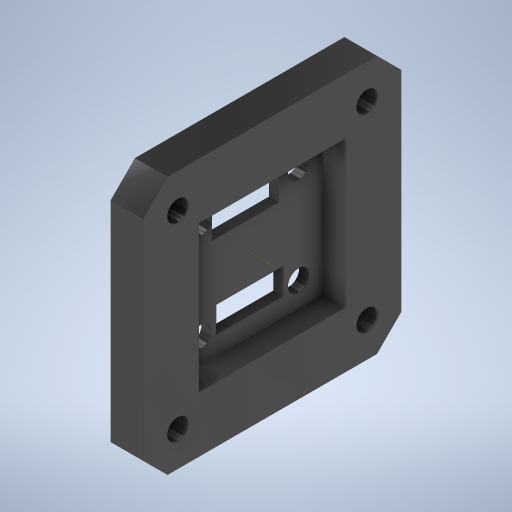
# Autodesk Inventor part: EncoderHalter
Saved by Autodesk Inventor 2023 (Build 270158000, 158)
## iProperties
Created: 2024-01-25
Part Number: EncoderHalter
Material: Generisch
Document SubType Name: Modeling
Designer: phili
Density: 1 g/cm^3
Appearance: Vorgabe
Author: phili
Autodesk Inventor part; units mm, degrees
ref_plane "YZ Plane" through (0, 0, 0) normal (1, 0, 0) x (0, 1, 0)
ref_plane "XZ Plane" through (0, 0, 0) normal (0, 1, 0) x (-1, 0, 0)
ref_plane "XY Plane" through (0, 0, 0) normal (0, 0, 1) x (1, 0, 0)
sketch "Skizze1" plane through (0, 0, 0) normal (1, 0, 0) x (0, 1, 0)
  line L0 (-21.15, -21.15) -> (21.15, -21.15)
  line L1 (21.15, -21.15) -> (21.15, 21.15)
  line L2 (21.15, 21.15) -> (-21.15, 21.15)
  line L3 (-21.15, 21.15) -> (-21.15, -21.15)
  line L4 (-21.15, -21.15) -> (21.15, 21.15) construction
  line L5 (21.15, -21.15) -> (-21.15, 21.15) construction
  point P0 (0, 0)
  dimension "d0" = 42.3
  dimension "d1" = 42.3
  constraints: 12 end point, 2 midpoint, 2 parallel, 1 horizontal, 1 perpendicular
  measures "d0" distance of L2.end L1.end
  measures "d1" distance of L1.end L0.end
extrude "Extrusion1" add sketch "Skizze1" along normal blind 5.3
sketch "Skizze2" plane through (5.3, 0, 0) normal (1, 0, 0) x (0, 0, -1)
  line L0 (12, -12) -> (-12, -12)
  line L1 (-12, -12) -> (-12, 12)
  line L2 (-12, 12) -> (12, 12)
  line L3 (12, 12) -> (12, -12)
  line L4 (12, -12) -> (-12, 12) construction
  line L5 (-12, -12) -> (12, 12) construction
  point P0 (0, 0)
  dimension "d4" = 24
  dimension "d5" = 24
  constraints: 12 end point, 2 midpoint, 2 parallel, 1 horizontal, 1 perpendicular
  measures "d4" distance of L1.end L2.end
  measures "d5" distance of L0.end L1.end
extrude "Extrusion2" cut sketch "Skizze2" against normal blind 3.7
sketch "Skizze3" plane through (1.6, 0, 0) normal (1, 0, 0) x (0, 0, -1)
  point P0 (0, 0)
  point P1 (-8, 8)
  point P2 (8, 8)
  point P3 (8, -8)
  point P4 (-8, -8)
  dimension "d16" = 8
  dimension "d17" = 8
  dimension "d18" = 8
  dimension "d19" = 8
  dimension "d20" = 8
  dimension "d21" = 8
  dimension "d22" = 8
  dimension "d23" = 8
  measures "d16" horizontal distance of point (0, 0) point (-8, 8)
  measures "d17" horizontal distance of point (0, 0) point (-8, -8)
  measures "d18" horizontal distance of point (0, 0) point (8, 8)
  measures "d19" horizontal distance of point (8, -8) point (0, 0)
  measures "d20" horizontal distance of point (0, 0) point (-8, -8)
  measures "d21" horizontal distance of point (8, -8) point (0, 0)
  measures "d22" horizontal distance of point (0, 0) point (-8, 8)
  measures "d23" horizontal distance of point (8, 8) point (0, 0)
hole "Bohrung1" at (1.6, 8, 8) at (1.6, 8, -8) at (1.6, -8, -8) at (1.6, -8, 8) direction (-1, 0, 0) diameter 3.5 end through all
sketch "Skizze4" plane through (5.3, 0, 0) normal (1, 0, 0) x (0, 0, -1)
  point P0 (0, 0)
  point P1 (-15.5, 15.5)
  point P2 (15.5, 15.5)
  point P3 (15.5, -15.5)
  point P4 (-15.5, -15.5)
  dimension "d31" = 15.5
  dimension "d32" = 15.5
  dimension "d33" = 15.5
  dimension "d34" = 15.5
  dimension "d35" = 15.5
  dimension "d36" = 15.5
  dimension "d37" = 15.5
  dimension "d38" = 15.5
  measures "d31" horizontal distance of point (0, 0) point (-15.5, 15.5)
  measures "d32" horizontal distance of point (0, 0) point (-15.5, 15.5)
  measures "d33" horizontal distance of point (15.5, 15.5) point (0, 0)
  measures "d34" horizontal distance of point (15.5, 15.5) point (0, 0)
  measures "d35" horizontal distance of point (15.5, -15.5) point (0, 0)
  measures "d36" horizontal distance of point (15.5, -15.5) point (0, 0)
  measures "d37" horizontal distance of point (0, 0) point (-15.5, -15.5)
  measures "d38" horizontal distance of point (-15.5, -15.5) point (0, 0)
hole "Bohrung2" at (5.3, 15.5, 15.5) at (5.3, 15.5, -15.5) at (5.3, -15.5, -15.5) at (5.3, -15.5, 15.5) direction (-1, 0, 0) diameter 3.4 end through all
chamfer "Fase1" distance 4 angle 45 4 edges at (2.65, -21.15, -21.15) (2.65, -21.15, 21.15) (2.65, 21.15, -21.15) (2.65, 21.15, 21.15)
sketch "Skizze5" plane through (1.6, 0, 0) normal (1, 0, 0) x (0, 0, -1)
  line L0 (-6.2, 9) -> (4.8, 9)
  line L1 (4.8, 9) -> (4.8, 4.7)
  line L2 (4.8, 4.7) -> (-6.2, 4.7)
  line L3 (-6.2, 4.7) -> (-6.2, 9)
  line L4 (-12, 12) -> (12, 12) projected
  line L5 (-12, -12) -> (-12, 12) projected
  point P0 (0, 0)
  point P1 (-6.2, 6.85)
  dimension "d42" = 11
  dimension "d43" = 4.3
  dimension "d44" = 3
  dimension "d45" = 5.8
  constraints: 8 end point, 2 parallel, 1 horizontal, 1 midpoint, 1 perpendicular
  measures "d42" distance of L1.end L2.end
  measures "d43" distance of L0.end L1.end
  measures "d44" distance between parallel lines of L4 L0
  measures "d45" distance from line of point (-6.2, 6.85) L5
sketch "Skizze6" plane through (1.6, 0, 0) normal (1, 0, 0) x (0, 0, -1)
  line L0 (-5.5, -4.7) -> (5.5, -4.7)
  line L1 (5.5, -4.7) -> (5.5, -9)
  line L2 (5.5, -9) -> (-5.5, -9)
  line L3 (-5.5, -9) -> (-5.5, -4.7)
  line L4 (12, -12) -> (-12, -12) projected
  point P0 (0, 0)
  dimension "d46" = 11
  dimension "d47" = 4.3
  dimension "d48" = 3
  dimension "d49" = 5.5
  constraints: 8 end point, 2 parallel, 1 horizontal, 1 perpendicular
  measures "d46" distance of L1.end L2.end
  measures "d47" distance of L0.end L1.end
  measures "d48" distance between parallel lines of L2 L4
  measures "d49" distance from line of point (0, 0) L3
extrude "Extrusion3" cut sketch "Skizze5" against normal blind 10
extrude "Extrusion4" cut sketch "Skizze6" against normal blind 10
